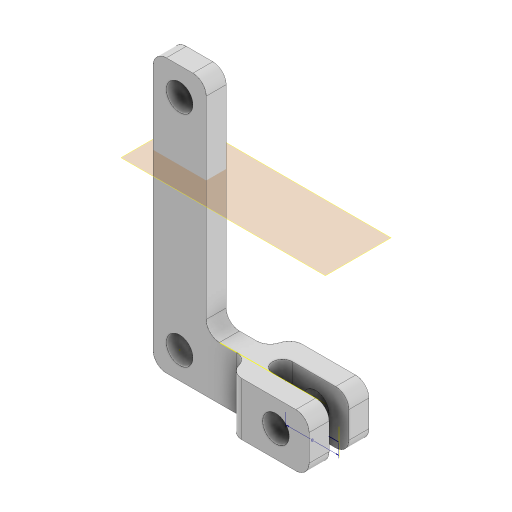
# Autodesk Inventor part: L_1
Saved by Autodesk Inventor 2023.5 (Build 275446020, 446B)
## iProperties
Created: 2025-07-10
Part Number: L_1
Material: Genérico
Document SubType Name: Modeling
Designer: jaime
Density: 1 g/cm^3
Appearance: Valor por defecto
Author: jaime
Autodesk Inventor part; units mm, degrees
ref_plane "YZ Plane" through (0, 0, 0) normal (1, 0, 0) x (0, 1, 0)
ref_plane "XZ Plane" through (0, 0, 0) normal (0, 1, 0) x (-1, 0, 0)
sketch "Boceto1" plane through (0, 0, 0) normal (0, 0, 1) x (1, 0, 0)
  circle A0 centre (0, 0) radius 2
  circle A1 centre (0, 33) radius 2
  line L0 (0, 0) -> (20, 0)
  line L1 (0, 0) -> (20, 0) construction
  circle A2 centre (20, 0) radius 2
  line L2 (0, -2) -> (0, -4)
  line L3 (0, -4) -> (24, -4)
  line L4 (24, -4) -> (24, 4)
  line L5 (24, 4) -> (4, 4)
  line L6 (4, 4) -> (4, 37)
  line L7 (4, 37) -> (-4, 37)
  line L8 (-4, 37) -> (-4, -4)
  line L9 (-4, -4) -> (0, -4)
  dimension "d0" = 4
  dimension "d2" = 20
  dimension "d3" = 0
  dimension "d4" = 4
  dimension "d5" = 2
  dimension "d6" = 24
  dimension "d7" = 8
  dimension "d8" = 20
  dimension "d10" = 8
  dimension "d11" = 33
  constraints: 20 end point, 6 perpendicular, 3 horizontal, 2 centre point, 2 coincident, 1 collinear, 1 point on line, 1 vertical, 1 vertical alignment, 2 other
  measures "d2" distance of L0.start L0.end
  measures "d3" distance between parallel lines of L0 L1
  measures "d4" diameter of A2
  measures "d5" distance of L2.start L2.end
  measures "d6" distance of L2.end L3.end
  measures "d7" distance of L3.end L4.end
  measures "d8" distance of L4.end L5.end
  measures "d10" distance of L6.end L7.end
  measures "d11" distance of point (0, 0) A1.centre
extrude "Extrusión1" add sketch "Boceto1" along normal blind 3
fillet "Empalme1" radius 2 6 edges at (-4, -4, 1.5) (24, -4, 1.5) (-4, 37, 1.5) (4, 37, 1.5) (4, 4, 1.5) (24, 4, 1.5)
sketch "Boceto2" plane through (4, 6, 0) normal (1, 0, 0) x (0, 0, -1)
  line L0 (-3, 29) -> (-3, 31) projected
  line L1 (-3, 31) -> (-3, 23)
  line L2 (-3, 25) -> (-3, 29) projected
  line L3 (-6, 23) -> (-6, 31)
  line L4 (-6, 31) -> (-3, 31)
  line L5 (3, 23) -> (3, 31)
  line L6 (3, 31) -> (0, 31)
  line L7 (0, 31) -> (0, 23)
  line L8 (0, 0) -> (0, 29) projected
  line L9 (-3, 25) -> (-3, 20)
  line L10 (-3, 0) -> (-3, 29) projected
  line L11 (-3, 20) -> (-6, 20)
  line L12 (-6, 20) -> (-6, 23)
  line L13 (0, 23) -> (0, 20)
  line L14 (3, 23) -> (3, 20)
  line L15 (3, 20) -> (0, 20)
  point P0 (0, -6)
  dimension "d18" = 5
  constraints: 24 end point, 5 perpendicular, 2 collinear, 2 point on line, 1 vertical
  measures "d18" distance of L2.start L9.end
extrude "Extrusión2" add sketch "Boceto2" against normal blind 8
fillet "Empalme2" radius 2 4 edges at (-4, 37, 4.5) (-4, 37, -1.5) (4, 37, 4.5) (4, 37, -1.5)
sketch "Boceto3" plane through (4, 26, 6) normal (0, 0, 1) x (1, 0, 0)
  circle A0 centre (-4, 7) radius 2 projected
  circle A1 centre (-4, 7) radius 2
  point P0 (-4, -26)
  constraints: 1 centre point, 1 coincident
extrude "Extrusión3" cut sketch "Boceto3" against normal through all
fillet "Empalme3" radius 2 4 edges at (0, 26, 6) (0, 26, 3) (0, 26, -3) (0, 26, 0)
sketch "Boceto4" plane through (-4, -2, 0) normal (-1, 0, 0) x (0, 0, 1)
  line L0 (6, 39) -> (-3, 39) projected
  line L1 (1.5, 39) -> (1.5, 30)
  line L2 (0, 30) -> (3, 30)
  line L3 (3, 30) -> (3, 39)
  line L4 (3, 39) -> (0, 39)
  line L5 (0, 39) -> (0, 30)
  line L6 (0, 30) -> (3, 39) construction
  line L7 (3, 30) -> (0, 39) construction
  point P0 (0, 2)
  point P1 (1.5, 34.5)
  dimension "d25" = 9
  dimension "d26" = 3
  constraints: 14 end point, 4 midpoint, 2 parallel, 1 horizontal, 1 perpendicular, 1 point on line, 1 vertical
  measures "d25" distance of L1.start L1.end
  measures "d26" distance of L4.end L3.end
extrude "Extrusión4" cut sketch "Boceto4" against normal blind 10
sketch "Boceto5" plane through (-4, -2, 0) normal (-1, 0, 0) x (0, 0, 1)
  point P0 (0, 2)
fillet "Empalme4" radius 1.5 2 edges at (0, 28, 0) (0, 28, 3)
ref_plane "Plano de trabajo1" through (4, 24.127, 3) normal (0, 1, 0) x (1, 0, 0)
sketch "Boceto6" plane through (0, 0, 3) normal (0, 0, 1) x (1, 0, 0)
  line L0 (24, -2) -> (24, 2) projected
  line L1 (24, 0) -> (16, 0)
  line L2 (22, 4) -> (6, 4) projected
  line L3 (16, 4) -> (16, -4.0705)
  point P0 (0, 0)
  dimension "d31" = 8
  constraints: 4 end point, 1 horizontal, 1 midpoint, 1 point on line, 1 vertical
  measures "d31" distance of L1.start L1.end
ref_plane "Plano de trabajo2" through (16, 4, 3) normal (1, 0, 0) x (0, -1, 0)
sketch "Boceto11" plane through (-2, -4, 0) normal (0, -1, 0) x (1, 0, 0)
  line L0 (24, 3) -> (8, 3) projected
  line L1 (20, 3) -> (20, 0) projected
  line L2 (24, 3) -> (20, 3)
  line L3 (17.5, 3) -> (17.5, 0)
  line L4 (20, 0) -> (24, 0)
  line L5 (20, 3) -> (15, 3)
  line L6 (15, 3) -> (15, 0)
  line L7 (24, 0) -> (8, 0) projected
  line L8 (20, 0) -> (15, 0)
  line L9 (26, 0) -> (26, 3) projected
  line L10 (20, 3) -> (26, 3)
  line L11 (26, 3) -> (26, 0)
  line L12 (26, 0) -> (20, 0)
  line L13 (20, 0) -> (20, 3)
  line L14 (15, 1.5) -> (16, 1.5)
  line L15 (15, 1.5) -> (16, 1.5)
  ellipse E0 centre (17.5, 1.5) end of major axis (17.5, 0) minor radius 1.5
  point P0 (2, 0)
  point P1 (17.5, 3)
  dimension "d44" = 5
  constraints: 24 end point, 3 parallel, 3 perpendicular, 2 horizontal, 2 midpoint, 2 point on line, 1 collinear, 1 vertical, 4 other
  measures "d44" distance of L5.start L5.end
extrude "Extrusión7" cut sketch "Boceto11" against normal blind 41 contours L10 L9 L12 L4 L1 L0 | L1 L7 E0 L0 | E0 L3 | L3 E0
sketch "Boceto12" plane through (-2, -4, 0) normal (0, -1, 0) x (1, 0, 0)
  line L0 (24, 3) -> (8, 3) projected
  line L1 (17.5, 3) -> (12.5, 3)
  line L2 (12.5, 3) -> (12.5, 0)
  line L3 (12.5, 0) -> (17.5, 0)
  line L4 (17.5, 0) -> (17.5, 3)
  line L5 (12.5, 3) -> (24.5, 3)
  line L6 (24.5, 3) -> (24.5, 6)
  line L7 (24.5, 6) -> (12.5, 6)
  line L8 (12.5, 6) -> (12.5, 3)
  line L9 (12.5, 0) -> (24.5, 0)
  line L10 (24.5, 0) -> (24.5, -3)
  line L11 (24.5, -3) -> (12.5, -3)
  line L12 (12.5, -3) -> (12.5, 0)
  point P0 (2, 0)
  point P1 (12.5, 3)
  dimension "d47" = 5
  dimension "d48" = 3
  dimension "d49" = 12
  dimension "d50" = 3
  dimension "d51" = 12
  dimension "d52" = 3
  constraints: 24 end point, 6 parallel, 3 horizontal, 3 perpendicular
  measures "d47" distance of L3.end L2.end
  measures "d48" distance of L2.end L1.end
  measures "d49" distance of L7.end L6.end
  measures "d50" distance of L6.end L5.end
  measures "d51" distance of L10.end L11.end
  measures "d52" distance of L9.end L10.end
extrude "Extrusión8" add sketch "Boceto12" against normal blind 8 contours L0 L8 L7 L6 L5 | L9 L10 L11 L12 L3
fillet "Empalme5" radius 2 8 edges at (22.5, 4, 4.5) (22.5, 4, -1.5) (22.5, -4, -1.5) (22.5, -4, 4.5) (10.5, 0, 3) (10.5, 0, 6) (10.5, 0, -3) (10.5, 0, 0)
sketch "Boceto13" plane through (20.5, -4, -3) normal (0, 0, -1) x (-1, 0, 0)
  line L0 (-2, 2) -> (-2, 6) projected
  line L1 (-2, 4) -> (3, 4)
  circle A0 centre (3, 4) radius 2
  point P0 (20.5, 4)
  dimension "d56" = 5
  dimension "d57" = 4
  constraints: 2 end point, 1 centre point, 1 coincident, 1 horizontal, 1 midpoint
  measures "d56" distance of L1.start L1.end
  measures "d57" diameter of A0
extrude "Extrusión9" cut sketch "Boceto13" against normal blind 100
sketch "Boceto14" plane through (-2, -4, 0) normal (0, -1, 0) x (1, 0, 0)
  arc A0 (17.5, 3) -> (17.5, 0) centre (17.5, 1.5) ccw projected
  line L0 (17.5, 1.5) -> (14.5, 1.5)
  line L1 (17.5, 3) -> (14.5, 3)
  line L2 (14.5, 3) -> (14.5, 0)
  circle A1 centre (16, 1.5) radius 1.5
  line L3 (14.5, 0) -> (17.5, 0)
  line L4 (17.5, 0) -> (21.5, 0) projected
  line L5 (17.5, 3) -> (17.5, 0)
  point P0 (2, 0)
  point P1 (16, 3)
  point P2 (16, 0)
  dimension "d60" = 3
  constraints: 10 end point, 3 horizontal, 2 perpendicular, 1 centre point, 1 midpoint
  measures "d60" distance of L0.start L0.end
extrude "Extrusión10" cut sketch "Boceto14" against normal through all contours A0 A1 L1 | A0 L0 A1 | A0 A1 L0 | A0 L3 A1 picked at (15.0125, 1.6113) picked at (15.0125, 1.3887)
split "Dividir3" plane through (4, 24.127, 3) removes the side toward (0, 1, 0)
sketch "Boceto15" plane through (0, 0, 3) normal (0, 0, 1) x (1, 0, 0)
  circle A0 centre (0, 0) radius 2 projected
  line L0 (0, 0) -> (0, 33)
  circle A1 centre (0, 33) radius 2
  line L1 (-4, 24.127) -> (-4, -2) projected
  line L2 (-4, 24.127) -> (4, 24.127)
  line L3 (4, 24.127) -> (4, 37.127)
  line L4 (4, 37.127) -> (-4, 37.127)
  line L5 (-4, 37.127) -> (-4, 24.127)
  dimension "d63" = 33
  dimension "d64" = 4
  dimension "d65" = 8
  dimension "d66" = 13
  constraints: 10 end point, 2 parallel, 1 centre point, 1 coincident, 1 horizontal, 1 perpendicular, 1 vertical
  measures "d63" distance of L0.start L0.end
  measures "d64" diameter of A1
  measures "d65" distance of L4.end L3.end
  measures "d66" distance of L3.end L2.end
extrude "Extrusión11" add sketch "Boceto15" against normal blind 3 contours L5 L4 L3 L2
fillet "Empalme6" radius 2 2 edges at (-4, 37.127, 1.5) (4, 37.127, 1.5)
